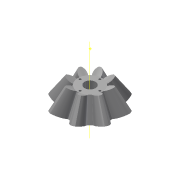
# Autodesk Inventor part: Bevel Gear1
Saved by Autodesk Inventor 2018 (Build 220112000, 112)
## iProperties
Created: 2018-08-06
Part Number: Bevel Gear1
Material: Steel, Mild
Document SubType Name: Modeling
Designer: Bardo91
Categories: <?xml version="1.0" encoding="UTF-16"?> <MemberInstance><Categories><FamilyTemplate><FamilyTemplateParameter ValueType="xs:double" Id="1" ObjectReferenceKey="da_z" ObjectType="kUserParameterObject"/><FamilyTemplateParameter ValueType="xs:double" Id="2" ObjectReferenceKey="da_b" ObjectType="kUserParameterObject"/><FamilyTemplateParameter ValueType="xs:double" Id="3" ObjectReferenceKey="da_beta" ObjectType="kUserParameterObject"/><FamilyTemplateParameter ValueType="xs:double" Id="4" ObjectReferenceKey="da_dae" ObjectType="kUserParameterObject"/><FamilyTemplateParameter ValueType="xs:double" Id="5" ObjectReferenceKey="da_ve" ObjectType="kUserParameterObject"/><FamilyTemplateParameter ValueType="xs:double" Id="6" ObjectReferenceKey="da_omega" ObjectType="kUserParameterObject"/><FamilyTemplateParameter ValueType="xs:string" Id="7" ObjectReferenceKey="EAIAABAAAAAAHwAAAAAAAIAAAAAAAAAA" ObjectType="83914240" SubObjectId="SurfaceGeometry"/></FamilyTemplate><ParamToTemplateMap><ParamToTemplate CategoryParameter="//CategoryParameter[@InternalName='046C89C9-8512-4d59-83FE-43B91F4F132A']" TemplateParameter="1"/><ParamToTemplate CategoryParameter="//CategoryParameter[@InternalName='2552DF32-E462-4b46-AEBF-C6C7768E72AC']" TemplateParameter="2"/><ParamToTemplate CategoryParameter="//CategoryParameter[@InternalName='C9EE641D-15FC-4fae-A226-E94C4372FDD7']" TemplateParameter="3"/><ParamToTemplate><ParamToTemplate CategoryParameter="//CategoryParameter[@InternalName='00B6519A-459B-49c7-AD84-2E56D39A5744']" ConstantValue="0.350000"/></ParamToTemplate><ParamToTemplate><ParamToTemplate CategoryParameter="//CategoryParameter[@InternalName='04B31F0E-C7A6-4894-AA32-9629BEFACF47']" ConstantValue="1.000000"/></ParamToTemplate><ParamToTemplate><ParamToTemplate CategoryParameter="//CategoryParameter[@InternalName='43CBEC2E-7847-49e7-A936-2F7889FCB2D9']" ConstantValue="0.200000"/></ParamToTemplate><ParamToTemplate><ParamToTemplate CategoryParameter="//CategoryParameter[@InternalName='B1EFC894-105D-4ebd-86BF-FA20ED196853']" ConstantValue="0.300000"/></ParamToTemplate><ParamToTemplate><ParamToTemplate CategoryParameter="//CategoryParameter[@InternalName='51175063-3D10-4879-93E8-6246FE8B403D']" ConstantValue="2060000000.000000"/></ParamToTemplate><ParamToTemplate><ParamToTemplate CategoryParameter="//CategoryParameter[@InternalName='A3A52E27-4454-46a9-B0BD-C932399B70AF']" ConstantValue="0.300000"/></ParamToTemplate><ParamToTemplate CategoryParameter="//CategoryParameter[@InternalName='2A200944-5A8C-41ca-B96E-8520D2E510F1']" TemplateParameter="4"/><ParamToTemplate><ParamToTemplate CategoryParameter="//CategoryParameter[@InternalName='1A637F62-92C8-44bc-B81F-10802510B579']" ConstantValue="1.703284"/></ParamToTemplate><ParamToTemplate CategoryParameter="//CategoryParameter[@InternalName='B52DD4BE-6863-48fb-BF58-89EF6F9EC65C']" TemplateParameter="5"/><ParamToTemplate><ParamToTemplate CategoryParameter="//CategoryParameter[@InternalName='3956BFF2-84D2-457d-93C2-9B0613DEBA67']" ConstantValue="1.256145"/></ParamToTemplate><ParamToTemplate CategoryParameter="//CategoryParameter[@InternalName='739CFA02-461B-4bf8-8049-181FCAD8B28F']" TemplateParameter="6"/><ParamToTemplate><ParamToTemplate CategoryParameter="//CategoryParameter[@InternalName='A27E999F-E2CE-4481-8A2A-EBF499C4C3C5']" ConstantValue="0.000000"/></ParamToTemplate><ParamToTemplate><ParamToTemplate CategoryParameter="//CategoryParameter[@InternalName='9E1B4470-B2D3-4ff1-B813-535BB4CDF51A']" ConstantValue="3520000.000000"/></ParamToTemplate><ParamToTemplate><ParamToTemplate CategoryParameter="//CategoryParameter[@InternalName='F8452263-BFF6-458c-9FB1-07C4B99E95CD']" ConstantValue="11400000.000000"/></ParamToTemplate><ParamToTemplate><ParamToTemplate CategoryParameter="//CategoryParameter[@InternalName='3E3BB259-FD49-497f-8171-6EBC954A3479']" ConstantValue="2.000000"/></ParamToTemplate><ParamToTemplate CategoryParameter="//CategoryParameter[@InternalName='27C3BAF2-7550-4e4b-AE2C-0DB134B7D9B7']" TemplateParameter="7"/></ParamToTemplateMap><Category DisplayName="Gear" InternalName="DC85795E-93AB-48d5-8EEE-5A27447B64BD" Mnemonic="Gear"><CategoryParameter DisplayName="z" InternalName="046C89C9-8512-4d59-83FE-43B91F4F132A" Mnemonic="z"/><CategoryParameter DisplayName="b" InternalName="2552DF32-E462-4b46-AEBF-C6C7768E72AC" Mnemonic="b"/><CategoryParameter DisplayName="||b|" InternalName="C9EE641D-15FC-4fae-A226-E94C4372FDD7" Mnemonic="beta"/><CategoryParameter DisplayName="x" InternalName="00B6519A-459B-49c7-AD84-2E56D39A5744" Mnemonic="x"/><CategoryParameter DisplayName="a*" InternalName="04B31F0E-C7A6-4894-AA32-9629BEFACF47" Mnemonic="a"/><CategoryParameter DisplayName="c*" InternalName="43CBEC2E-7847-49e7-A936-2F7889FCB2D9" Mnemonic="c"/><CategoryParameter DisplayName="r|.f|*" InternalName="B1EFC894-105D-4ebd-86BF-FA20ED196853" Mnemonic="rf"/><CategoryParameter DisplayName="E" InternalName="51175063-3D10-4879-93E8-6246FE8B403D" Mnemonic="E"/><CategoryParameter DisplayName="||m|" InternalName="A3A52E27-4454-46a9-B0BD-C932399B70AF" Mnemonic="mi"/><Category DisplayName="BevelGear" InternalName="0C98F69A-0C2B-4791-B2FE-7691BB227E77" Mnemonic="BevelGear"><CategoryParameter DisplayName="d|.ae|" InternalName="2A200944-5A8C-41ca-B96E-8520D2E510F1" Mnemonic="dae"/><CategoryParameter DisplayName="d|.ai|" InternalName="1A637F62-92C8-44bc-B81F-10802510B579" Mnemonic="dai"/><CategoryParameter DisplayName="A|.e|" InternalName="B52DD4BE-6863-48fb-BF58-89EF6F9EC65C" Mnemonic="ve"/><CategoryParameter DisplayName="A|.i|" InternalName="3956BFF2-84D2-457d-93C2-9B0613DEBA67" Mnemonic="vi"/><CategoryParameter DisplayName="||S|" InternalName="739CFA02-461B-4bf8-8049-181FCAD8B28F" Mnemonic="omega"/><CategoryParameter DisplayName="x|.t|" InternalName="A27E999F-E2CE-4481-8A2A-EBF499C4C3C5" Mnemonic="xt"/><CategoryParameter DisplayName="||s||.Flim|" InternalName="9E1B4470-B2D3-4ff1-B813-535BB4CDF51A" Mnemonic="sFlim"/><CategoryParameter DisplayName="||s||.Hlim|" InternalName="F8452263-BFF6-458c-9FB1-07C4B99E95CD" Mnemonic="sHlim"/><CategoryParameter DisplayName="type" InternalName="3E3BB259-FD49-497f-8171-6EBC954A3479" Mnemonic="type"/><CategoryParameter DisplayName="PitchDiameter" InternalName="27C3BAF2-7550-4e4b-AE2C-0DB134B7D9B7" Mnemonic="IDS_PITCHDIAM"/></Category></Category></Categories></MemberInstance>
Mass: 60.9118 g
Surface Area: 34.3074 cm^2
Volume: 7.7496 cm^3
Density: 7.86 g/cm^3
Appearance: Steel
CustomPartVersion: 1
Author: Bardo91
Autodesk Inventor part; units mm, degrees
ref_plane "Mesh Plane2" through (0, 0, 0) normal (0.9238795, 0.3826834, 0) x (0, 0, 1)
sketch "Teeth Body Sketch" plane through (0, 0, 0) normal (1, 0, 0) x (0, 1, 0)
  line L0 (0, 0) -> (9.071263, -23.464368) construction
  line L1 (9.071263, -23.464368) -> (14.17744, -20.91128)
  line L2 (14.17744, -20.91128) -> (0, 0) construction
  line L3 (11.2, -22.4) -> (0, 0) construction
  line L4 (5.449127, -14.095096) -> (8.516419, -12.561451)
  line L5 (9.071263, -23.464368) -> (5.449127, -14.095096)
  line L6 (14.17744, -20.91128) -> (8.516419, -12.561451)
  line L7 (0, -39.386751) -> (0, 6.564458)
  line L8 (0, -22.4) -> (14.17744, -22.4) construction
  dimension "d0" = 22.4
  dimension "d1" = 18.14253
  dimension "d2" = 28.35488
  dimension "d3" = 10
  dimension "d4" = 20.91128
  constraints: 16 end point, 4 point on line, 3 perpendicular, 2 collinear, 1 horizontal alignment, 1 vertical alignment
  measures "d0" diameter of L3.start L7
  measures "d1" diameter of L0.end L7
  measures "d2" diameter of L1.end L7
  measures "d3" distance between parallel lines of L1 L4
  measures "d4" vertical distance of L1.end L0.start
revolve "Teeth Body" add sketch "Teeth Body Sketch" angle 360 about axis through (0, 0, 0) along (0, 0, 1)
ref_plane "Tooth Plane" through (0, 11.2, -22.4) normal (0, -0.4472136, 0.8944272) x (1, 0, 0)
sketch "Start Sketch" plane through (0, 11.2, -22.4) normal (0, -0.4472136, 0.8944272) x (1, 0, 0)
  line L0 (0, -23.505131) -> (0, 10.644758)
  arc A0 (-0.89083, -3.065065) -> (-7.690533, 3.268304) centre (-7.631558, -3.48525) ccw
  arc A1 (7.690533, 3.268304) -> (0.89083, -3.065065) centre (7.631558, -3.48525) ccw
  line L1 (-0.89083, -3.065065) -> (0.89083, -3.065065)
  arc A2 (7.690533, 3.268304) -> (-7.690533, 3.268304) centre (0, -12.521981) ccw
  dimension "d7" = 6.75381
  dimension "d8" = 7.63156
  dimension "d9" = 9.03673
  dimension "d57" = 17.56352
  dimension "d58" = 9.45692
  constraints: 6 point on circle, 3 centre point, 3 symmetric about line, 2 end point, 1 coincident, 1 perpendicular, 1 other
  measures "d7" radius of A0
  measures "d8" horizontal distance of point (0, -12.522) A0.centre
  measures "d9" vertical distance of point (0, -12.522) A0.centre
  measures "d57" radius of A2
  measures "d58" distance from line of A2.centre L1
sketch "End Sketch" plane through (0, 6.60021, -13.200419) normal (0, -0.4472136, 0.8944272) x (1, 0, 0)
  line L0 (0, -15.358918) -> (0, 6.982715)
  arc A0 (-0.525861, -1.7968) -> (-4.539756, 1.941816) centre (-4.504942, -2.044837) ccw
  arc A1 (4.539756, 1.941816) -> (0.525861, -1.7968) centre (4.504942, -2.044837) ccw
  line L1 (-0.525861, -1.7968) -> (0.525861, -1.7968)
  arc A2 (4.539756, 1.941816) -> (-4.539756, 1.941816) centre (0, -7.379259) ccw
  dimension "d12" = 3.9868
  dimension "d15" = 4.50494
  dimension "d16" = 5.33442
  dimension "d59" = 10.36783
  dimension "d60" = 5.58246
  constraints: 6 point on circle, 3 centre point, 3 symmetric about line, 2 end point, 1 coincident, 1 other
  measures "d12" radius of A0
  measures "d15" horizontal distance of A0.centre point (0, -7.379)
  measures "d16" vertical distance of A0.centre point (0, -7.379)
  measures "d59" radius of A2
  measures "d60" distance from line of A2.centre L1
loft "Loft" cut profiles "Start Sketch", "End Sketch"
pattern_circular "Circular Pattern" count 8 over 360 about axis through (0, 0, 0) along (0, 0, 1) of "Loft"
ref_plane "End Plane" through (0, 6.60021, -13.200419) normal (0, -0.4472136, 0.8944272) x (1, 0, 0)
sketch3d "3D Sketch Right"
ref_plane "End Plane Right" through (-2.677006, 6.032943, -13.200419) normal (0.1813872, -0.4087771, 0.8944272) x (0.9140533, 0.4055941, 0)
sketch "End Sketch Right" plane through (-2.677006, 6.032943, -13.200419) normal (0.1813872, -0.4087771, 0.8944272) x (0.9140533, 0.4055941, 0)
  arc A0 (-0.525861, -1.7968) -> (-4.539756, 1.941816) centre (-4.504942, -2.044837) ccw
  line L0 (0, -21.485512) -> (0, 13.109297)
  arc A1 (4.539756, 1.941816) -> (0.525861, -1.7968) centre (4.504942, -2.044837) ccw
  line L1 (-0.525861, -1.7968) -> (0.525861, -1.7968)
  arc A2 (4.539756, 1.941816) -> (-4.539756, 1.941816) centre (0, -7.379259) ccw
  dimension "d70" = 4.50494
  dimension "d71" = 5.33442
  dimension "d72" = 3.9868
  dimension "d73" = 5.58246
  dimension "d74" = 10.36783
  constraints: 6 point on circle, 3 centre point, 3 symmetric about line, 2 end point, 1 coincident, 1 perpendicular, 1 other
  measures "d70" horizontal distance of A2.centre A0.centre
  measures "d71" vertical distance of point (0, -7.379) A0.centre
  measures "d72" radius of A0
  measures "d73" distance from line of point (0, -7.379) L1
  measures "d74" radius of A2
feature "Loft Right" [suppressed]
pattern_circular "Circular Pattern Right" [suppressed]
sketch3d "3D Sketch Left"
ref_plane "End Plane Left" through (2.620563, 6.032943, -13.184182) normal (-0.17786, -0.4094614, 0.8948225) x (0.9172065, -0.3984121, 0)
sketch "End Sketch Left" plane through (2.620563, 6.032943, -13.184182) normal (-0.17786, -0.4094614, 0.8948225) x (0.9172065, -0.3984121, 0)
  line L0 (0, -37.747693) -> (0, 20.749362)
  arc A0 (-0.525861, -1.783741) -> (-4.539756, 1.954874) centre (-4.504942, -2.031778) ccw
  arc A1 (4.539756, 1.954874) -> (0.525861, -1.783741) centre (4.504942, -2.031778) ccw
  line L1 (-0.525861, -1.783741) -> (0.525861, -1.783741)
  ellipse E0 centre (0, -5.607711) end of major axis (8.516419, -5.607711) minor radius 7.620683
  arc A2 (4.539756, 1.954874) -> (-4.539756, 1.954874) centre (0, -7.3662) ccw
  dimension "d56" = 7.62068
  dimension "d30" = 3.9868
  dimension "d31" = 4.50494
  dimension "d32" = 5.33442
  dimension "d61" = 10.36783
  dimension "d62" = 5.58246
  constraints: 6 point on circle, 3 centre point, 3 symmetric about line, 2 end point, 1 coincident, 2 other
  measures "d30" radius of A0
  measures "d31" horizontal distance of point (0, -7.366) A0.centre
  measures "d32" vertical distance of A0.centre point (0, -7.366)
  measures "d61" radius of A2
  measures "d62" distance from line of point (0, -7.366) L1
feature "Loft Left" [suppressed]
pattern_circular "Circular Pattern Left" [suppressed]
sketch "Body Sketch" plane through (0, 0, 0) normal (1, 0, 0) x (0, 1, 0)
  line L0 (0, -35.037536) -> (0, -19.530831)
  line L1 (9.071263, -23.464368) -> (5.449127, -14.095096)
  line L2 (5.449127, -14.095096) -> (0, -14.095096)
  line L3 (9.071263, -23.464368) -> (0, -23.464368)
  constraints: 4 end point, 2 perpendicular, 2 point on line
sketch "Body Sketch outline for Fix Body" plane through (0, 0, 0) normal (1, 0, 0) x (0, 1, 0)
  line L0 (0, -23.464368) -> (9.071263, -23.464368)
  line L1 (0, -14.095096) -> (0, -23.464368)
  line L2 (5.449127, -14.095096) -> (0, -14.095096)
  line L3 (9.071263, -23.464368) -> (5.449127, -14.095096)
revolve "Fix Body" add sketch "Body Sketch outline for Fix Body" angle 360 about axis through (0, 0, 0) along (0, 0, 1)
sketch "Sketch6" plane through (0, 0, 0) normal (1, 0, 0) x (0, 1, 0)
  line L0 (11.2, -22.4) -> (0, 0)
  line L1 (0, -37.799919) -> (0, 6.299986)
surface revolve "Pitch Diameter" sketch "Sketch6" angle 360 about axis through (0, 0, 0) along (0, 0, 1) shown no curves L0
sketch "Sketch8" plane through (0, 0, -14.095096) normal (0, 0, 1) x (1, 0, 0)
  circle A0 centre (0, 0) radius 2.5
  dimension "d94" = 5
  constraints: 1 centre point, 1 coincident
  measures "d94" diameter of A0
extrude "Extrusion1" cut sketch "Sketch8" against normal through all
sketch "Sketch9" plane through (0, 0, -23.464368) normal (0, 0, -1) x (-1, 0, 0)
  line L0 (0, 0) -> (0, 4.5)
  circle A0 centre (0, 4.5) radius 0.5
  circle A1 centre (-4.5, 0) radius 0.5
  circle A2 centre (0, -4.5) radius 0.5
  circle A3 centre (4.5, 0) radius 0.5
  dimension "d97" = 4.5
  dimension "d98" = 1
  dimension "d101" = 360
  constraints: 4 centre point, 2 end point, 1 coincident, 1 vertical, 9 other
  measures "d97" distance of L0.start L0.end
  measures "d98" diameter of A0
extrude "Extrusion2" cut sketch "Sketch9" against normal through all
equation "\"d0\" = da_de"
equation "\"d1\" = da_dfe"
equation "\"d2\" = da_dae"
equation "\"d3\" = da_b"
equation "\"d4\" = da_ve"
equation "\"d7\" = fd_rr"
equation "\"d8\" = fd_x"
equation "\"d9\" = fd_y"
equation "\"d57\" = 0.5 * fd_dva + 0.3 * da_he"
equation "\"d58\" = 0.5 * fd_dva - 1.12 * da_he"
equation "\"da_teethtype\" = 0"
equation "\"da_b\" = 10"
equation "\"da_de\" = 22.4"
equation "\"da_dae\" = 28.35488"
equation "\"da_dfe\" = 18.14253"
equation "\"da_le\" = 25.04396"
equation "\"da_omega\" = 90deg"
equation "\"da_beta\" = 0"
equation "\"da_delta\" = 26.565051deg"
equation "\"da_alpha\" = 20deg"
equation "\"da_he\" = 5.70888"
equation "\"da_ve\" = 20.91128"
equation "\"da_zv\" = 8.944272"
equation "\"fd_loft\" = da_b + 0.05 * da_he"
equation "\"fd_x\" = fd_x1 + fd_x2"
equation "\"fd_y\" = fd_y1 - fd_y2"
equation "\"fd_dd\" = fd_dva - 0.8 * da_he"
equation "\"da_dvw\" = 27.00396"
equation "\"d11\" = fd_loft"
equation "\"da_dm\" = 17.92786"
equation "\"da_x\" = 0.35"
equation "\"da_m\" = 2.8"
equation "\"d50\" = da_omega"
equation "\"fd_rr\" = 6.753811"
equation "\"fd_dva\" = 31.70172"
equation "\"fd_x1\" = 2.38499"
equation "\"fd_x2\" = 5.246568"
equation "\"fd_y1\" = 13.289669"
equation "\"fd_y2\" = 4.252939"
body "Solid1"
body "Srf1"
